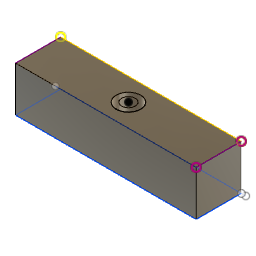
Bearing Arm hole (Autodesk Fusion 360 design; units mm, degrees)
Autodesk Fusion 360 part; units mm, degrees
sketch "Top" plane through (0, 0, 0) normal (0, 0, 1) x (1, 0, 0)
  line L0 (80, -110) -> (37.8078, -110)
  line L1 (79, -110) -> (79, -120)
  line L2 (79, -120) -> (39, -120)
  line L3 (39, -120) -> (39, -110)
  dimension "d29" = 40
  dimension "d30" = 10
  dimension "d31" = 1
  constraint vertical L1
  constraint horizontal L2
  constraint vertical L3
  constraint coincident L0 L3.end
  measures "d29" distance of L3.end L1.start
  measures "d30" distance of L3.end L2.end
  measures "d31" distance of L0.start L1.start
extrude "Extrude2" add sketch "Top" along normal blind 10
sketch "Sketch3" plane through (0, 0, 10) normal (0, 0, 1) x (-1, 0, 0)
  line L0 (-79, 110) -> (-39, 110)
  line L1 (-39, 120) -> (-79, 120)
  circle A0 centre (-59, 115) radius 1.5
  circle A1 centre (-59, 115) radius 2.7
  line L2 (-39, 110) -> (-79, 110)
  line L3 (-79, 110) -> (-79, 120)
  line L4 (-79, 120) -> (-79, 110)
  line L5 (-39, 110) -> (-39, 120)
  dimension "d49" = 3
  dimension "d52" = 5.4
  dimension "d55" = 5
  dimension "d57" = 20
  constraint concentric A0 A1
  measures "d49" diameter of A0
  measures "d52" diameter of A1
  measures "d55" distance of A0.centre L2
  measures "d57" distance of A0.centre L3
extrude "Extrude9" cut sketch "Sketch3" against normal blind 4 contours A1
extrude "Extrude8" cut sketch "Sketch3" against normal blind 100 contours A0
equation "wheel_hub_point_width = 60 mm"
equation "chassis_point_full_length = wheel_hub_point_width + ( wheel_hub_point_width / 2 )"
equation "thickness = 10 mm"
equation "length = 100 mm"
equation "d13 = thickness"
equation "extra = 100 mm"
equation "hub_width = 40 mm"
equation "d29 = hub_width"
equation "d30 = thickness"
equation "chassis_point_gap = 56.8 mm"
equation "chassis_points_length = 16.6 mm"
equation "bearing_682ZZ_outer_radius = 2.7 mm"
equation "bearing_big_distance = hub_width / 2"
equation "bearing_small_distance = thickness / 2"
equation "bearing_682ZZ_inner_radius = 1.5 mm"
equation "bearing_682ZZ_width = 4 mm"
equation "d49 = bearing_682ZZ_inner_radius * 2"
equation "d50 = -extra"
equation "d52 = bearing_682ZZ_outer_radius * 2"
equation "d53 = -bearing_682ZZ_width"
equation "d55 = bearing_small_distance"
equation "d57 = bearing_big_distance"
